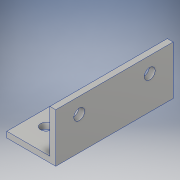
# Autodesk Inventor part: Mounting Bracket
Saved by Autodesk Inventor 2019.4 (Build 234330000, 330)
## iProperties
Created: 2020-01-24
Part Number: Mounting Bracket
Material: Aluminum 6061
Document SubType Name: Modeling
Designer: admin
Density: 2.7 g/cm^3
Appearance: Aluminum - Flat
Mass: 18.2652 g
Surface Area: 52.9928 cm^2
Volume: 6.7649 cm^3
Author: admin
Autodesk Inventor part; units mm, degrees
ref_plane "YZ Plane" through (0, 0, 0) normal (1, 0, 0) x (0, 1, 0)
ref_plane "XZ Plane" through (0, 0, 0) normal (0, 1, 0) x (-1, 0, 0)
ref_plane "XY Plane" through (0, 0, 0) normal (0, 0, 1) x (1, 0, 0)
sketch "Sketch1" plane through (0, 0, 0) normal (0, 0, 1) x (1, 0, 0)
  line L0 (0, 0) -> (-25, 0)
  line L1 (-25, 0) -> (-25, 3)
  line L2 (-25, 3) -> (-3, 3)
  line L3 (-3, 3) -> (-3, 25)
  line L4 (-3, 25) -> (0, 25)
  line L5 (0, 25) -> (0, 0)
  dimension "d0" = 3
  dimension "d1" = 3
  dimension "d2" = 25
  dimension "d3" = 25
  constraints: 12 end point, 5 perpendicular, 1 horizontal
  measures "d0" distance between parallel lines of L0 L2
  measures "d1" distance between parallel lines of L5 L3
  measures "d2" distance of L0.start L0.end
  measures "d3" distance of L4.end L0.start
extrude "Extrusion1" add sketch "Sketch1" along normal blind 60
sketch "Sketch2" plane through (-25, 3, 0) normal (0, 1, 0) x (1, 0, 0)
  circle A0 centre (8, -48) radius 2.75
  circle A1 centre (8, -12) radius 2.75
  line L0 (8, -48) -> (8, -12) construction
  line L1 (8, -30) -> (0, -30) construction
  line L2 (0, 0) -> (0, -60) projected
  circle A2 centre (8, -30) radius 2.75
  point P0 (25, 0)
  dimension "d6" = 5.5
  dimension "d7" = 5.5
  dimension "d8" = 8
  dimension "d9" = 36
  dimension "d12" = 5.5
  constraints: 4 end point, 3 centre point, 2 midpoint, 1 coincident, 1 perpendicular, 1 vertical
  measures "d6" diameter of A0
  measures "d7" diameter of A1
  measures "d8" distance of L1.start L1.end
  measures "d9" distance of L0.start L0.end
  measures "d12" diameter of A2
extrude "Extrusion2" cut sketch "Sketch2" against normal through all contours A0 | A1
ref_plane "Work Plane1" through (-3, 3, 0) normal (0.7071068, 0.7071068, 0) x (0, 0, 1)
mirror "Mirror1" about plane through (-3, 3, 0) normal (0.7071068, 0.7071068, 0) of "Extrusion2"
body "Solid1"
